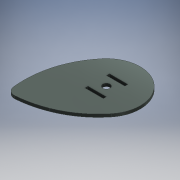
# Autodesk Inventor part: leva00
Saved by Autodesk Inventor 2016 (Build 200138000, 138)
## iProperties
Created: 2016-09-20
Part Number: leva00
Material: Madera (abedul)
Document SubType Name: Modeling
Designer: i95sa
Density: 0.55 g/cm^3
Appearance: Gris plomo - Pulido
Author: i95sa
Autodesk Inventor part; units mm, degrees
ref_plane "YZ Plane" through (0, 0, 0) normal (1, 0, 0) x (0, 1, 0)
ref_plane "XZ Plane" through (0, 0, 0) normal (0, 1, 0) x (-1, 0, 0)
ref_plane "XY Plane" through (0, 0, 0) normal (0, 0, 1) x (1, 0, 0)
sketch "Boceto1" plane through (0, 0, 0) normal (0, 0, 1) x (1, 0, 0)
  arc A0 (29.2514, 35.3589) -> (-29.2514, -35.3589) centre (0, 0) ccw
  arc A1 (-45.0156, -54.4145) -> (-58.5162, -70.734) centre (-51.7659, -62.5742) ccw
  line L0 (-60.4706, -73.0964) -> (-68.6303, -66.3461)
  line L1 (-35.0099, 29.6682) -> (-48.6094, 40.9187)
  line L2 (-48.6094, 40.9187) -> (-68.6303, -66.3461)
  line L3 (-68.6303, -66.3461) -> (-60.8581, -24.7052)
  arc A2 (-35.0099, 29.6682) -> (-60.8581, -24.7052) centre (54.5789, -46.2515) ccw
  arc A3 (-60.8581, -24.7052) -> (-62.2905, -63.7493) centre (69.4964, -49.0358) ccw
  line L4 (2.2501, 2.7199) -> (29.2514, 35.3589)
  line L5 (-2.2501, -2.7199) -> (-60.4706, -73.0964)
  arc A4 (-29.2514, -35.3589) -> (29.2514, 35.3589) centre (0, 0) ccw
  arc A5 (-58.5162, -70.734) -> (-45.0156, -54.4145) centre (-51.7659, -62.5742) ccw
  line L6 (-60.4706, -73.0964) -> (-52.3109, -79.8467)
  line L7 (35.7029, -28.8305) -> (49.3024, -40.081)
  line L8 (49.3024, -40.081) -> (-52.3109, -79.8467)
  line L9 (-52.3109, -79.8467) -> (-12.864, -64.4094)
  arc A6 (-12.864, -64.4094) -> (35.7029, -28.8305) centre (-55.6593, 44.9455) ccw
  arc A7 (-50.948, -73.1326) -> (-12.864, -64.4094) centre (-61.1896, 59.0771) ccw
  dimension "d0" = 91.78
  dimension "d6" = 21.18
  dimension "d7" = 10.59
  dimension "d8" = 17.65
  dimension "d9" = 42.36
  constraints: 20 end point, 20 point on circle, 8 centre point, 6 symmetric about line, 5 point on line, 4 tangent, 1 collinear, 4 other
  measures "d0" diameter of A0
  measures "d6" diameter of A1
  measures "d7" distance of L0.start L0.end
  measures "d8" distance of L1.start L1.end
  measures "d9" distance of L0.end L3.end
extrude "Extrusión2" add sketch "Boceto1" along normal blind 4 contours A4 A0 | A0 L5 A1 A3 A2 | A6 A7 A5 L5 A4 | L5 A1 | A5 L5
sketch "Boceto2" plane through (0, 0, 4) normal (0, 0, 1) x (1, 0, 0)
  line L0 (0, 0) -> (0, 12.5)
  line L1 (0, 12.5) -> (-12.5, 12.5)
  line L2 (-12.5, 12.5) -> (-12.5, 16.7)
  line L3 (-12.5, 16.7) -> (12.5, 16.7)
  line L4 (12.5, 16.7) -> (12.5, 12.5)
  line L5 (12.5, 12.5) -> (0, 12.5)
  line L6 (0, 0) -> (12.5, 0)
  line L7 (0, 0) -> (0, -12.5)
  line L8 (0, -12.5) -> (-12.5, -12.5)
  line L9 (-12.5, -12.5) -> (-12.5, -16.7)
  line L10 (-12.5, -16.7) -> (12.5, -16.7)
  line L11 (12.5, -16.7) -> (12.5, -12.5)
  line L12 (12.5, -12.5) -> (0, -12.5)
  circle A0 centre (0, 0) radius 5
  dimension "d24" = 12.5
  dimension "d25" = 12.5
  dimension "d26" = 4.2
  dimension "d27" = 25
  dimension "d28" = 10
  constraints: 26 end point, 5 perpendicular, 5 symmetric about line, 3 point on line, 1 centre point, 1 coincident, 1 parallel, 1 vertical
  measures "d24" distance of L0.start L0.end
  measures "d25" distance of L0.end L1.end
  measures "d26" distance of L1.end L2.end
  measures "d27" distance of L2.end L3.end
  measures "d28" diameter of A0
extrude "Extrusión3" cut sketch "Boceto2" against normal blind 4
